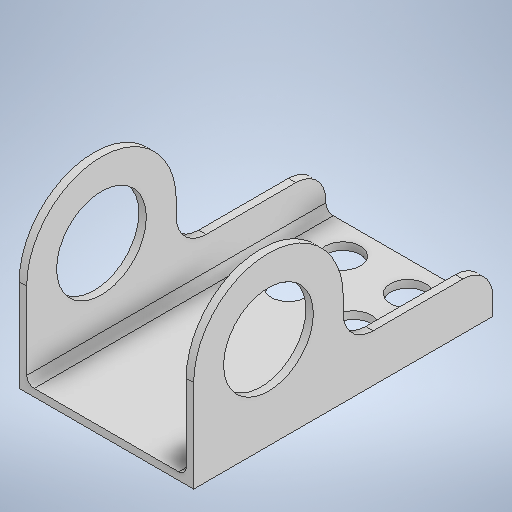
# Autodesk Inventor part: whateverthisis
Saved by Autodesk Inventor 2025 (Build 290162000, 162)
## iProperties
Created: 2025-04-26
Part Number: whateverthisis
Material: Všeobecné
Document SubType Name: Modeling
Designer: jakub
Density: 1 g/cm^3
Appearance: Výchozí
Author: jakub
Autodesk Inventor part; units mm, degrees
ref_plane "YZ Plane" through (0, 0, 0) normal (1, 0, 0) x (0, 1, 0)
ref_plane "XZ Plane" through (0, 0, 0) normal (0, 1, 0) x (-1, 0, 0)
ref_plane "XY Plane" through (0, 0, 0) normal (0, 0, 1) x (1, 0, 0)
sketch "Sketch1" plane through (0, 0, 0) normal (0, 1, 0) x (-1, 0, 0)
  line L0 (0, 0) -> (-70, 0)
  line L1 (-70, 0) -> (-70, -120)
  line L2 (-70, -120) -> (0, -120)
  line L3 (0, -120) -> (0, 0)
  line L4 (0, -120) -> (-3, -120)
  line L5 (-3, -120) -> (-3, 0)
  line L6 (-70, 0) -> (-67, 0)
  line L7 (-67, 0) -> (-67, -120)
  dimension "d0" = 70
  dimension "d1" = 120
  dimension "d2" = 3
  dimension "d3" = 3
  constraints: 16 end point, 4 point on line, 3 perpendicular, 2 parallel, 1 horizontal
  measures "d0" distance of L2.end L1.end
  measures "d1" distance of L1.end L0.end
  measures "d2" distance of L2.end L4.end
  measures "d3" distance of L0.end L6.end
extrude "Extrusion1" add sketch "Sketch1" along normal blind 3
sketch "Sketch2" plane through (0, 3, 0) normal (0, 1, 0) x (1, 0, 0)
  line L0 (70, 0) -> (70, 120) projected
  line L1 (70, 120) -> (0, 120)
  line L2 (0, 120) -> (0, 0)
  line L3 (0, 0) -> (70, 0)
  line L4 (70, 0) -> (70, 120)
  line L5 (70, 120) -> (67, 120)
  line L6 (67, 120) -> (67, 0)
  line L7 (0, 0) -> (3, 0)
  line L8 (3, 0) -> (3, 120)
  dimension "d6" = 3
  dimension "d7" = 3
  constraints: 16 end point, 4 point on line, 3 perpendicular, 2 parallel, 1 horizontal
  measures "d6" distance of L0.end L5.end
  measures "d7" distance of L2.end L7.end
extrude "Extrusion2" add sketch "Sketch2" along normal blind 70 contours L3 L6 L1 L0 | L3 L2 L1 L8
sketch "Sketch3" plane through (0, 0, -120) normal (-1, 0, 0) x (0, 0, 1)
  line L0 (120, 0) -> (90, 0)
  line L1 (90, 0) -> (120, 0)
  line L2 (90, 0) -> (127, 0)
  line L3 (120, 0) -> (0, 0) projected
  line L4 (90, 0) -> (90, 37)
  circle A0 centre (90, 37) radius 18
  circle A1 centre (90, 37) radius 30
  line L5 (0, 0) -> (0, 7)
  line L6 (0, 3) -> (0, 73) projected
  line L7 (12, 19) -> (48, 19)
  arc A2 (12, 19) -> (0, 7) centre (12, 7) ccw
  line L8 (60, 37) -> (60, 31)
  arc A3 (48, 19) -> (60, 31) centre (48, 31) ccw
  line L9 (0, 7) -> (0, 73)
  line L10 (0, 73) -> (120, 73)
  line L11 (120, 73) -> (120, 37)
  point P0 (0, 19)
  point P1 (66, 19)
  dimension "d10" = 30
  dimension "d12" = 37
  dimension "d13" = 36
  dimension "d14" = 60
  dimension "d15" = 19
  dimension "d16" = 12
  dimension "d17" = 12
  constraints: 20 end point, 8 point on circle, 6 tangent, 5 point on line, 4 centre point, 3 collinear, 3 horizontal, 2 coincident, 2 perpendicular, 1 vertical
  measures "d10" distance of L0.start L0.end
  measures "d12" distance of L0.end L4.end
  measures "d13" diameter of A0
  measures "d14" diameter of A1
  measures "d15" distance of L3.end point (0, 19)
  measures "d16" radius of A2
  measures "d17" radius of A3
extrude "Extrusion3" cut sketch "Sketch3" against normal blind 70 contours L8 A3 L7 A2 L6 L10 L11 A1
sketch "Sketch4" plane through (0, 0, -120) normal (-1, 0, 0) x (0, 0, 1)
  line L0 (120, 0) -> (90, 0)
  line L1 (0, 0) -> (120, 0) projected
  line L2 (90, 0) -> (90, 37)
  circle A0 centre (90, 37) radius 18
  dimension "d20" = 30
  dimension "d21" = 37
  dimension "d22" = 36
  constraints: 4 end point, 1 centre point, 1 coincident, 1 point on line, 1 vertical
  measures "d20" distance of L0.start L0.end
  measures "d21" distance of L0.end L2.end
  measures "d22" diameter of A0
extrude "Extrusion4" cut sketch "Sketch4" against normal blind 70
fillet "Fillet1" radius 3 2 edges at (3, 3, -60) (67, 3, -60)
sketch "Sketch5" plane through (0, 3, 0) normal (0, 1, 0) x (1, 0, 0)
  line L0 (67, 0) -> (67, 120) projected
  line L1 (67, 120) -> (56, 120)
  line L2 (70, 120) -> (0, 120) projected
  line L3 (3, 120) -> (3, 0) projected
  line L4 (3, 120) -> (5.3284, 120)
  line L5 (3, 120) -> (14, 120)
  circle A0 centre (48.0638, 86.1207) radius 7
  circle A1 centre (48.0638, 107.9241) radius 7
  circle A2 centre (21.9362, 86.1207) radius 7
  circle A3 centre (21.9362, 107.9241) radius 7
  point P0 (0, 0)
  constraints: 6 end point, 4 centre point, 3 point on line
extrude "Extrusion5" cut sketch "Sketch5" against normal blind 70
body "Solid1"
